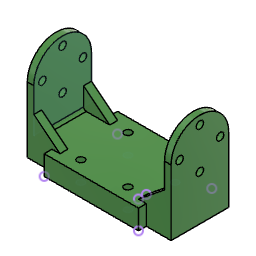
Servo Base Bracket v4 (Autodesk Fusion 360 design; units mm, degrees)
Autodesk Fusion 360 part; units mm, degrees
sketch "Servo Bracket" plane through (0, 0, 0) normal (0, 1, 0) x (1, 0, 0)
  line L0 (18, 11) -> (27.45, 11)
  line L1 (18, -14) -> (-18, -14)
  line L2 (27.45, -11) -> (27.45, 11)
  line L3 (-27.45, 11) -> (-18, 11)
  line L4 (-18, -14) -> (-18, -11)
  circle A0 centre (-9, 9) radius 1.5 construction
  line L5 (18, -11) -> (18, -14)
  circle A1 centre (9, 9) radius 1.5 construction
  line L6 (-18, 11) -> (-18, 14)
  line L7 (-18, 14) -> (18, 14)
  line L8 (27.45, -11) -> (18, -11)
  circle A2 centre (9, -9) radius 1.5 construction
  line L9 (18, 14) -> (18, 11)
  circle A3 centre (-9, -9) radius 1.5 construction
  line L10 (-18, -11) -> (-27.45, -11)
  line L11 (-27.45, 11) -> (-27.45, -11)
  line L12 (9, 9) -> (-9, 9) construction
  line L13 (-9, 9) -> (-9, -9) construction
  line L14 (-9, -9) -> (9, -9) construction
  line L15 (9, -9) -> (9, 9) construction
  line L16 (9, 9) -> (-9, -9) construction
  line L17 (-9, 9) -> (9, -9) construction
  point P0 (-27.45, 0)
  point P1 (0, 14)
  dimension "d1" = 22
  dimension "d2" = 36
  dimension "d3" = 3
  dimension "d4" = 27.45
  dimension "d5" = 27.45
  dimension "d6" = 9.45
  dimension "d7" = 3
  constraint equal L5 L9
  constraint equal L4 L6
  constraint equal L2 L11
  constraint horizontal L7
  constraint horizontal L1
  constraint vertical L2
  constraint vertical L11
  constraint midpoint L11 P0
  constraint horizontal origin P0
  constraint midpoint L7 P1
  constraint vertical origin P1
  constraint equal L0 L3
  constraint equal L3 L10
  constraint equal L0 L8
  constraint horizontal L12
  constraint perpendicular L12 L13
  constraint parallel L12 L14
  constraint parallel L13 L15
  constraint coincident A1.centre L12.start
  constraint coincident L16 origin
  constraint coincident L17 origin
  measures "d1" distance of L2.start L0.end
  measures "d3" distance of L1.start L5.start
  measures "d4" horizontal distance of L2.start origin
  measures "d5" horizontal distance of L10.end origin
  measures "d6" distance of L3.end L3.start
  measures "d7" diameter of A1
extrude "Extrude1" add sketch "Servo Bracket" along normal blind 2.5
sketch "Sketch2" plane through (0, 2.5, 0) normal (0, 1, 0) x (-1, 0, 0)
  line L0 (-9, -9) -> (9, -9) construction
  line L1 (9, -9) -> (9, 9) construction
  line L2 (9, 9) -> (-9, 9) construction
  line L3 (-9, 9) -> (-9, -9) construction
  line L4 (-9, -9) -> (9, 9) construction
  line L5 (9, -9) -> (-9, 9) construction
  point P0 (9, -9)
  point P1 (-9, -9)
  point P2 (-9, 9)
  point P3 (9, 9)
  dimension "d10" = 18
  constraint horizontal L0
  constraint perpendicular L0 L1
  constraint parallel L0 L2
  constraint parallel L1 L3
  constraint coincident L4 origin
  constraint coincident L5 origin
  constraint equal L0 L3
  constraint coincident P0 L0.end
  constraint coincident L0.start L3.end
  constraint coincident P2 L2.end
  constraint coincident L1.end L2.start
  measures "d10" distance of L0.start P2
hole "Hole1" at (9, 2.5, -9) at (-9, 2.5, -9) at (-9, 2.5, 9) at (9, 2.5, 9) direction (0, -1, 0) diameter 2.8 depth 3 tip angle 180
sketch "Sketch3" plane through (0, 2.5, 0) normal (0, 1, 0) x (-1, 0, 0)
  line L0 (-27.45, 11) -> (-27.45, -11)
  line L1 (27.45, -11) -> (27.45, 11)
  line L2 (-27.45, 11) -> (-24.95, 11)
  line L3 (-24.95, 11) -> (-24.95, -11)
  line L4 (-24.95, -11) -> (-27.45, -11)
  line L5 (-27.45, -11) -> (-27.45, 11)
  line L6 (27.45, 11) -> (24.95, 11)
  line L7 (24.95, 11) -> (24.95, -11)
  line L8 (24.95, -11) -> (27.45, -11)
  line L9 (27.45, -11) -> (27.45, 11)
  dimension "d14" = 2.5
  dimension "d15" = 2.5
  constraint horizontal L2
  constraint vertical L3
  constraint horizontal L4
  constraint vertical L5
  constraint coincident L0.start L2.start
  constraint horizontal L6
  constraint vertical L7
  constraint horizontal L8
  constraint vertical L9
  constraint coincident L1.end L6.start
  constraint coincident L0.end L4.end
  constraint coincident L1.start L8.end
  measures "d14" distance of L3.end L0.end
  measures "d15" distance of L7.end L1.start
extrude "Extrude2" add sketch "Sketch3" along normal blind 28.5
fillet "Fillet1" radius 11 4 edges at (26.2, 31, 11) (26.2, 31, -11) (-26.2, 31, -11) (-26.2, 31, 11)
sketch "Sketch4" plane through (27.45, 0, 0) normal (1, 0, 0) x (0, 0, -1)
  arc A0 (11, 20) -> (-11, 20) centre (0, 20) ccw construction
  circle A1 centre (0, 20) radius 7.75 construction
  point P0 (7.75, 20.0171)
  point P1 (0, 27.75)
  point P2 (-7.75, 20.0171)
  point P3 (0, 12.25)
  dimension "d19" = 15.5
  constraint concentric A0 A1
  constraint coincident A1 P0
  constraint coincident A1 P1
  constraint coincident A1 P2
  constraint coincident A1 P3
  measures "d19" diameter of A1
hole "Hole2" at (27.45, 27.75, 0) at (27.45, 20.0171, 7.75) at (27.45, 20.0171, -7.75) at (27.45, 12.25, 0) direction (-1, 0, 0) diameter 2.8 depth 3 tip angle 180
mirror "Mirror1" about plane through (0, 0, 0) normal (1, 0, 0) of "Hole2"
sketch "Sketch5" plane through (0, 2.5, 0) normal (0, 1, 0) x (-1, 0, 0)
  circle A0 centre (0, 0) radius 2
  dimension "d25" = 4
  constraint coincident A0.centre origin
  measures "d25" diameter of A0
fillet "Fillet2" radius 1 2 edges at (-24.95, 2.5, 0) (24.95, 2.5, 0)
sketch "Sketch6" plane through (0, 0, 0) normal (0, -1, 0) x (1, 0, 0)
  line L0 (18, 14) -> (-18, 14)
  line L1 (-18, -14) -> (18, -14)
  circle A0 centre (9, -9) radius 1.4
  circle A1 centre (9, 9) radius 1.4
  circle A2 centre (-9, 9) radius 1.4
  circle A3 centre (-9, -9) radius 1.4
  line L2 (18, -14) -> (18, 14)
  line L3 (-18, -14) -> (-18, 14)
  constraint coincident L1.end L2.start
  constraint coincident L0.start L2.end
  constraint coincident L1.start L3.start
  constraint coincident L0.end L3.end
extrude "Extrude4" add sketch "Sketch6" along normal blind 2
sketch "草图8" plane through (0, -2, 0) normal (0, -1, 0) x (1, 0, 0)
  circle A0 centre (-9, -9) radius 1.4
  circle A1 centre (-9, 9) radius 1.4
  circle A2 centre (9, -9) radius 1.4
  circle A3 centre (9, 9) radius 1.4
  line L0 (18, -14) -> (18, 14)
  line L1 (18, 14) -> (-18, 14)
  line L2 (-18, 14) -> (-18, -14)
  line L3 (-18, -14) -> (18, -14)
extrude "拉伸6" add sketch "草图8" along normal blind 3
sketch "草图9" plane through (-24.95, 0, 0) normal (1, 0, 0) x (0, 0, -1)
  line L0 (-11, 3.5) -> (11, 3.5)
  line L1 (11, 3.5) -> (11, 20)
  arc A0 (11, 20) -> (-11, 20) centre (0, 20) ccw
  line L2 (-11, 20) -> (-11, 3.5)
  circle A1 centre (0, 12.25) radius 1.4
  circle A2 centre (-7.75, 20.0171) radius 1.4
  circle A3 centre (0, 27.75) radius 1.4
  circle A4 centre (7.75, 20.0171) radius 1.4
sketch "草图10" plane through (18, 0, 0) normal (1, 0, 0) x (0, 0, -1)
  line L0 (-11, 0) -> (-11, 2.5)
  line L1 (-11, 2.5) -> (-14, 2.5)
  line L2 (-14, 2.5) -> (-14, -5)
  line L3 (-14, -5) -> (14, -5)
  line L4 (14, -5) -> (14, 2.5)
  line L5 (14, 2.5) -> (11, 2.5)
  line L6 (11, 2.5) -> (11, 0)
  line L7 (11, 0) -> (-11, 0)
  line L8 (-11, 0) -> (-9, 0)
  line L9 (-9, 0) -> (-4, 0)
  line L10 (-4, 0) -> (-4, -3.5)
  line L11 (-4, -3.5) -> (-9, -3.5)
  line L12 (-9, -3.5) -> (-9, 0)
  line L13 (11, 0) -> (9.5, 0)
  line L14 (9.5, 0) -> (4.5, 0)
  line L15 (4.5, 0) -> (4.5, -3.5)
  line L16 (4.5, -3.5) -> (9.5, -3.5)
  line L17 (9.5, -3.5) -> (9.5, 0)
  dimension "d41" = 5
  dimension "d42" = 3.5
  dimension "d43" = 1.5
  dimension "d44" = 5
  dimension "d45" = 3.5
  constraint coincident L0.start L7.end
  constraint coincident L7 L8.end
  constraint perpendicular L0 L8
  constraint horizontal L9
  constraint vertical L10
  constraint horizontal L11
  constraint vertical L12
  constraint coincident L6.end L7.start
  constraint perpendicular L6 L13
  constraint horizontal L14
  constraint vertical L15
  constraint horizontal L16
  constraint vertical L17
  measures "d41" distance of L8.end L9.end
  measures "d42" distance of L8.end L11.end
  measures "d43" distance of L6.end L13.end
  measures "d44" distance of L13.end L14.end
  measures "d45" distance of L13.end L16.end
extrude "拉伸7" add sketch "草图10" along normal blind 4 contours L7 L9 L10 L11 L12 | L7 L14 L15 L16 L17
sketch "草图11" plane through (0, 0, 9) normal (0, 0, 1) x (1, 0, 0)
  line L0 (18, 0) -> (18, -3.5)
  line L1 (18, -3.5) -> (22, -3.5)
  line L2 (22, -3.5) -> (22, 0)
  line L3 (22, 0) -> (18, 0)
  line L4 (22, 0) -> (18, -3.5)
  constraint coincident L2.end L3.start
  constraint coincident L0.end L1.start
extrude "拉伸8" cut sketch "草图11" against normal blind 5 contours L1 L2 L4
sketch "草图12" plane through (0, 0, -9.5) normal (0, 0, -1) x (-1, 0, 0)
  line L0 (-18, -3.5) -> (-18, 0)
  line L1 (-18, 0) -> (-22, 0)
  line L2 (-22, 0) -> (-22, -3.5)
  line L3 (-22, -3.5) -> (-18, -3.5)
  line L4 (-22, 0) -> (-18, -3.5)
  constraint coincident L1.end L2.start
  constraint coincident L0.start L3.end
extrude "拉伸9" cut sketch "草图12" against normal blind 5 contours L2 L3 L4
sketch "草图13" plane through (-18, 0, 0) normal (-1, 0, 0) x (0, 0, 1)
  line L0 (14, -5) -> (14, 2.5)
  line L1 (14, 2.5) -> (11, 2.5)
  line L2 (11, 2.5) -> (11, 0)
  line L3 (11, 0) -> (-11, 0)
  line L4 (-11, 0) -> (-11, 2.5)
  line L5 (-11, 2.5) -> (-14, 2.5)
  line L6 (-14, 2.5) -> (-14, -5)
  line L7 (-14, -5) -> (14, -5)
  line L8 (-11, 0) -> (-9.5, 0)
  line L9 (-9.5, 0) -> (-4.5, 0)
  line L10 (-4.5, 0) -> (-4.5, -3.5)
  line L11 (-4.5, -3.5) -> (-9.5, -3.5)
  line L12 (-9.5, -3.5) -> (-9.5, 0)
  line L13 (11, 0) -> (9.5, 0)
  line L14 (9.5, 0) -> (4.5, 0)
  line L15 (4.5, 0) -> (4.5, -3.5)
  line L16 (4.5, -3.5) -> (9.5, -3.5)
  line L17 (9.5, -3.5) -> (9.5, 0)
  dimension "d52" = 1.5
  dimension "d53" = 5
  dimension "d54" = 3.5
  dimension "d55" = 1.5
  dimension "d56" = 5
  dimension "d57" = 3.5
  constraint coincident L3.end L4.start
  constraint perpendicular L4 L8
  constraint horizontal L9
  constraint vertical L10
  constraint horizontal L11
  constraint vertical L12
  constraint coincident L2.end L3.start
  constraint coincident L3 L13.end
  constraint horizontal L14
  constraint vertical L15
  constraint horizontal L16
  constraint vertical L17
  measures "d52" distance of L3.end L8.end
  measures "d53" distance of L8.end L9.end
  measures "d54" distance of L8.end L11.end
  measures "d55" distance of L2.end L13.end
  measures "d56" distance of L13.end L14.end
  measures "d57" distance of L13.end L16.end
extrude "拉伸10" add sketch "草图13" along normal blind 4 contours L3 L14 L15 L16 L17 | L3 L9 L10 L11 L12
sketch "草图14" plane through (0, 0, 9.5) normal (0, 0, 1) x (1, 0, 0)
  line L0 (-18, -3.5) -> (-18, 0)
  line L1 (-18, 0) -> (-22, 0)
  line L2 (-22, 0) -> (-22, -3.5)
  line L3 (-22, -3.5) -> (-18, -3.5)
  line L4 (-22, 0) -> (-18, -3.5)
  constraint coincident L1.end L2.start
  constraint coincident L0.start L3.end
extrude "拉伸11" cut sketch "草图14" against normal blind 5 contours L2 L3 L4
sketch "草图15" plane through (0, 0, -9.5) normal (0, 0, -1) x (-1, 0, 0)
  line L0 (18, 0) -> (18, -3.5)
  line L1 (18, -3.5) -> (22, -3.5)
  line L2 (22, -3.5) -> (22, 0)
  line L3 (22, 0) -> (18, 0)
  line L4 (18, -3.5) -> (22, 0)
  constraint coincident L0.end L1.start
  constraint coincident L2.end L3.start
extrude "拉伸12" cut sketch "草图15" against normal blind 5 contours L1 L2 L4
sketch "草图16" plane through (-24.95, 0, 0) normal (1, 0, 0) x (0, 0, -1)
sketch "草图17" plane through (-24.95, 0, 0) normal (1, 0, 0) x (0, 1, 0)
sketch "草图18" plane through (-24.95, 0, 0) normal (1, 0, 0) x (0, 0, -1)
  line L0 (11, 3.5) -> (11, 20)
  line L1 (11, 3.5) -> (11, 4)
  line L2 (11, 4) -> (11, 11.5)
  line L3 (11, 2.5, 3.975) -> (8, 2.5, 3.975)
  line L4 (8, 2.5, 3.975) -> (8, 10.5, 3.975)
  line L5 (8, 10.5, 3.975) -> (11, 10.5, 3.975)
  line L6 (11, 10.5, 3.975) -> (11, 2.5, 3.975)
  line L7 (11, 2.5, 6.95) -> (11, 2.5, 1)
  dimension "d67" = 3
  dimension "d68" = 8
  constraint coincident L0.start L1.start
  constraint coincident L0 L1.end
  constraint coincident L0 L2.end
extrude "拉伸13" cut sketch "草图18" against normal blind 5 contours L3 L4 L5 L6 in plane through (-20.975, 0, 0) normal (1, 0, 0)
sketch "草图19" plane through (-24.95, 0, 0) normal (1, 0, 0) x (0, 0, -1)
  line L0 (-11, 2.5, 3.975) -> (-8, 2.5, 3.975)
  line L1 (-8, 2.5, 3.975) -> (-8, 10.5, 3.975)
  line L2 (-8, 10.5, 3.975) -> (-11, 10.5, 3.975)
  line L3 (-11, 10.5, 3.975) -> (-11, 2.5, 3.975)
  line L4 (-11, 2.5, 1) -> (-11, 2.5, 6.95)
  dimension "d71" = 3
  dimension "d72" = 8
extrude "拉伸14" cut sketch "草图19" against normal blind 5 contours L0 L1 L2 L3 in plane through (-20.975, 0, 0) normal (1, 0, 0)
extrude "拉伸15" add 1 faces at (-25.975, 7.8333, 10) along direction (1, 0, 0) blind 11
sketch "草图20" plane through (0, 0, 11) normal (0, 0, 1) x (1, 0, 0)
  line L0 (-24.95, 10.5) -> (-24.95, 20)
  line L1 (-24.95, 20) -> (-27.45, 20)
  line L2 (-27.45, 20) -> (-27.45, 0)
  line L3 (-27.45, 0) -> (-18, 0)
  line L4 (-18, 0) -> (-18, 2.5)
  line L5 (-18, 2.5) -> (-14.975, 2.5)
  line L6 (-14.975, 2.5) -> (-14.975, 10.5)
  line L7 (-14.975, 10.5) -> (-24.95, 10.5)
  line L8 (-24.95, 10.5) -> (-14.975, 2.5)
  constraint coincident L0.start L7.end
  constraint coincident L5.end L6.start
extrude "拉伸16" cut sketch "草图20" against normal blind 3 contours L6 L7 L8
extrude "拉伸17" add 1 faces at (-25.975, 5.1667, -10) along direction (1, 0, 0) blind 11
sketch "草图21" plane through (0, 0, -11) normal (0, 0, -1) x (-1, 0, 0)
  line L0 (18, 2.5) -> (18, 0)
  line L1 (18, 0) -> (27.45, 0)
  line L2 (27.45, 0) -> (27.45, 20)
  line L3 (27.45, 20) -> (24.95, 20)
  line L4 (24.95, 20) -> (24.95, 10.5)
  line L5 (24.95, 10.5) -> (14.975, 10.5)
  line L6 (14.975, 10.5) -> (14.975, 2.5)
  line L7 (14.975, 2.5) -> (18, 2.5)
  line L8 (14.975, 2.5) -> (24.95, 10.5)
  constraint coincident L6.end L7.start
  constraint coincident L4.end L5.start
extrude "拉伸18" cut sketch "草图21" against normal blind 3 contours L5 L6 L8
sketch "草图22" plane through (24.95, 0, 0) normal (-1, 0, 0) x (0, 0, 1)
  line L0 (-11, 3.5) -> (11, 3.5)
  line L1 (11, 3.5) -> (11, 20)
  arc A0 (11, 20) -> (-11, 20) centre (0, 20) ccw
  line L2 (-11, 20) -> (-11, 3.5)
  circle A1 centre (0, 12.25) radius 1.4
  circle A2 centre (7.75, 20.0171) radius 1.4
  circle A3 centre (0, 27.75) radius 1.4
  circle A4 centre (-7.75, 20.0171) radius 1.4
  line L3 (11, 2.5, 3.975) -> (7.9516, 2.5, 3.975)
  line L4 (7.9516, 2.5, 3.975) -> (7.9516, 10.5, 3.975)
  line L5 (7.9516, 10.5, 3.975) -> (11, 10.5, 3.975)
  line L6 (11, 10.5, 3.975) -> (11, 2.5, 3.975)
  line L7 (11, 2.5, 6.95) -> (11, 2.5, 1)
  dimension "d83" = 8
extrude "拉伸19" cut sketch "草图22" against normal blind 5 contours L3 L4 L5 L6 in plane through (20.975, 0, 0) normal (-1, 0, 0)
sketch "草图23" plane through (24.95, 0, 0) normal (-1, 0, 0) x (0, 0, 1)
  line L0 (7.9516, 10.5) -> (11, 10.5)
  line L1 (11, 10.5) -> (11, 20)
  arc A0 (11, 20) -> (-11, 20) centre (0, 20) ccw
  line L2 (-11, 20) -> (-11, 3.5)
  line L3 (-11, 3.5) -> (7.9516, 3.5)
  line L4 (7.9516, 3.5) -> (7.9516, 10.5)
  circle A1 centre (0, 12.25) radius 1.4
  circle A2 centre (7.75, 20.0171) radius 1.4
  circle A3 centre (0, 27.75) radius 1.4
  circle A4 centre (-7.75, 20.0171) radius 1.4
  line L5 (-11, 2.5, 3.975) -> (-8, 2.5, 3.975)
  line L6 (-8, 2.5, 3.975) -> (-8, 10.5, 3.975)
  line L7 (-8, 10.5, 3.975) -> (-11, 10.5, 3.975)
  line L8 (-11, 10.5, 3.975) -> (-11, 2.5, 3.975)
  line L9 (-11, 2.5, 1) -> (-11, 2.5, 6.95)
  dimension "d86" = 3
  dimension "d87" = 8
extrude "拉伸20" cut sketch "草图23" against normal blind 5 contours L5 L6 L7 L8 in plane through (20.975, 0, 0) normal (-1, 0, 0)
extrude "拉伸21" add 1 faces at (25.975, 7.8333, -10) along direction (-1, 0, 0) blind 11
extrude "拉伸22" add 1 faces at (25.975, 5.1667, 9.9839) along direction (-1, 0, 0) blind 11
sketch "草图24" plane through (0, 0, 11) normal (0, 0, 1) x (1, 0, 0)
  line L0 (18, 2.5) -> (18, 0)
  line L1 (18, 0) -> (27.45, 0)
  line L2 (27.45, 0) -> (27.45, 20)
  line L3 (27.45, 20) -> (24.95, 20)
  line L4 (24.95, 20) -> (24.95, 10.5)
  line L5 (24.95, 10.5) -> (14.975, 10.5)
  line L6 (14.975, 10.5) -> (14.975, 2.5)
  line L7 (14.975, 2.5) -> (18, 2.5)
  line L8 (14.975, 2.5) -> (24.95, 10.5)
  constraint coincident L6.end L7.start
  constraint coincident L4.end L5.start
sketch "草图25" plane through (14.975, 0, 0) normal (-1, 0, 0) x (0, 0, 1)
  line L0 (7.9516, 2.5) -> (11, 2.5)
extrude "拉伸23" cut sketch "草图24" against normal blind 4 contours L5 L6 L8
sketch "草图26" plane through (0, 0, -11) normal (0, 0, -1) x (-1, 0, 0)
  line L0 (-24.95, 10.5) -> (-24.95, 20)
  line L1 (-24.95, 20) -> (-27.45, 20)
  line L2 (-27.45, 20) -> (-27.45, 0)
  line L3 (-27.45, 0) -> (-18, 0)
  line L4 (-18, 0) -> (-18, 2.5)
  line L5 (-18, 2.5) -> (-14.975, 2.5)
  line L6 (-14.975, 2.5) -> (-14.975, 10.5)
  line L7 (-14.975, 10.5) -> (-24.95, 10.5)
  line L8 (-24.95, 10.5) -> (-14.975, 2.5)
  constraint coincident L0.start L7.end
  constraint coincident L5.end L6.start
extrude "拉伸24" cut sketch "草图26" against normal blind 3 contours L6 L7 L8
sketch "草图27" plane through (0, -5, 0) normal (0, -1, 0) x (1, 0, 0)
  circle A0 centre (9, -9) radius 1.4
  circle A1 centre (-9, -9) radius 1.4
  circle A2 centre (-9, 9) radius 1.4
  circle A3 centre (9, 9) radius 1.4
  line L0 (-18, -14) -> (18, -14)
  line L1 (18, 14) -> (-18, 14)
extrude "拉伸25" cut 1 faces at (-19.3333, -1.1667, 9.5) along direction (0, 0, -1) blind 5
extrude "拉伸26" cut 1 faces at (-19.3333, -1.1667, -9.5) along direction (0, 0, 1) blind 5
extrude "拉伸27" cut 1 faces at (19.3333, -1.1667, 9) along direction (0, 0, -1) blind 5
extrude "拉伸28" cut 1 faces at (19.3333, -1.1667, -9.5) along direction (0, 0, 1) blind 5
extrude "拉伸29" add 3 faces at (25.6333, 0, 1.3333) (19.3333, 0, 7.3333) (19.3333, 0, -7.8333) along direction (0, -1, 0) blind 5
extrude "拉伸30" add 3 faces at (-25.6333, 0, -1.5) (-19.3333, 0, -7.8333) (-19.3333, 0, 7.8333) along direction (0, -1, 0) blind 5
sketch "Sketch7" plane through (0, 2.5, 0) normal (0, 1, 0) x (-1, 0, 0)
  circle A0 centre (9, 9) radius 1.4
  circle A1 centre (-9, 9) radius 1.4
  circle A2 centre (21.3705, 7.091) radius 2.75
  circle A3 centre (-21.3705, 7.091) radius 2.75
  line L0 (21.3705, 7.091) -> (-21.3705, 7.091) construction
  point P0 (0, 7.091)
  dimension "d31" = 5.5
  dimension "d32" = 1.909
  dimension "d33" = 42.741
  constraint equal A2 A3
  constraint horizontal A2.centre A3.centre
  constraint coincident A2.centre L0.start
  constraint coincident A3.centre L0.end
  constraint midpoint L0 P0
  constraint vertical origin P0
  measures "d31" diameter of A2
  measures "d32" vertical distance of A0.centre A2.centre
  measures "d33" distance of A2.centre A3.centre
extrude "Extrude5" [suppressed]
